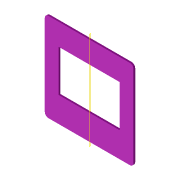
# Autodesk Inventor part: 00_Grating_1000linesPerMM
Saved by Autodesk Inventor 2022 (Build 260153000, 153)
## iProperties
Created: 2023-02-14
Part Number: 00_Grating_1000linesPerMM
Material: Generisch
Document SubType Name: Modeling
Designer: diederichbenedict
Density: 1 g/cm^3
Appearance: Glatt - Violett
Author: diederichbenedict
Autodesk Inventor part; units mm, degrees
ref_plane "YZ Plane" through (0, 0, 0) normal (1, 0, 0) x (0, 1, 0)
ref_plane "XZ Plane" through (0, 0, 0) normal (0, 1, 0) x (-1, 0, 0)
ref_plane "XY Plane" through (0, 0, 0) normal (0, 0, 1) x (1, 0, 0)
sketch "Skizze1" plane through (0, 0, 0) normal (0, 0, 1) x (1, 0, 0)
  line L0 (23.5, -25.5) -> (-23.5, -25.5)
  line L1 (-25.5, -23.5) -> (-25.5, 23.5)
  line L2 (-23.5, 25.5) -> (23.5, 25.5)
  line L3 (25.5, 23.5) -> (25.5, -23.5)
  line L4 (25.5, -25.5) -> (-25.5, 25.5) construction
  line L5 (-25.5, -25.5) -> (25.5, 25.5) construction
  line L6 (-17.5, 13) -> (17.5, 13)
  line L7 (17.5, 13) -> (17.5, -11)
  line L8 (17.5, -11) -> (-17.5, -11)
  line L9 (-17.5, -11) -> (-17.5, 13)
  line L10 (-17.5, 13) -> (17.5, -11) construction
  line L11 (17.5, 13) -> (-17.5, -11) construction
  arc A0 (-23.5, 25.5) -> (-25.5, 23.5) centre (-23.5, 23.5) ccw
  arc A1 (25.5, 23.5) -> (23.5, 25.5) centre (23.5, 23.5) ccw
  arc A2 (23.5, -25.5) -> (25.5, -23.5) centre (23.5, -23.5) ccw
  arc A3 (-25.5, -23.5) -> (-23.5, -25.5) centre (-23.5, -23.5) ccw
  point P0 (0, 0)
  point P1 (0, 1)
  dimension "d0" = 51
  dimension "d1" = 51
  dimension "d2" = 35
  dimension "d3" = 24
  dimension "d4" = 12.5
  dimension "d5" = 2
  constraints: 24 end point, 8 point on circle, 8 point on line, 8 tangent, 4 centre point, 4 midpoint, 4 parallel, 3 equal radius, 2 horizontal, 2 perpendicular
  measures "d0" distance of L4.end L5.end
  measures "d1" distance of L5.start L4.end
  measures "d2" distance of L7.end L8.end
  measures "d3" distance of L6.end L7.end
  measures "d4" distance between parallel lines of L6 L2
  measures "d5" radius of A0
extrude "Extrusion1" add sketch "Skizze1" along normal blind 1
ref_plane "Arbeitsebene1" through (0, -23.5, 0) normal (1, 0, 0) x (0, 0, -1)
